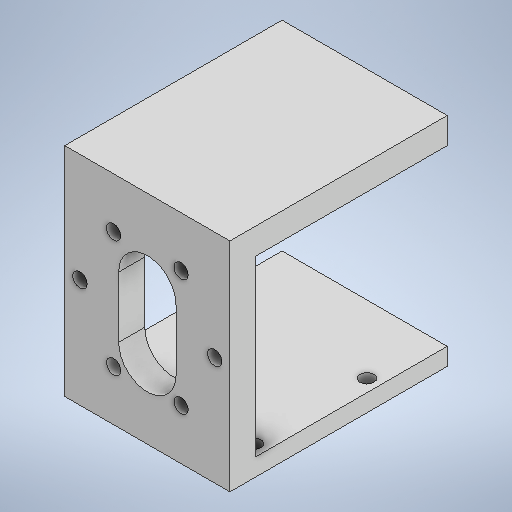
# Autodesk Inventor part: ギアボックス
Saved by Autodesk Inventor 2026.2 (Build 302298010, 298A)
## iProperties
Created: 2026-05-06
Part Number: ギアボックス
Material: 一般
Document SubType Name: Modeling
Designer: Yagis
Density: 1 g/cm^3
Appearance: 既定
Author: Yagis
Autodesk Inventor part; units mm, degrees
ref_plane "YZ Plane" through (0, 0, 0) normal (1, 0, 0) x (0, 1, 0)
ref_plane "XZ Plane" through (0, 0, 0) normal (0, 1, 0) x (-1, 0, 0)
ref_plane "XY Plane" through (0, 0, 0) normal (0, 0, 1) x (1, 0, 0)
sketch "スケッチ1" plane through (0, 0, 0) normal (0, 0, 1) x (1, 0, 0)
  line L0 (0, 0) -> (38, 0)
  line L1 (38, 0) -> (38, 24)
  line L2 (38, 24) -> (0, 24)
  line L3 (0, 24) -> (0, 0)
  line L4 (0, 4) -> (38, 4)
  line L5 (12.4, 31) -> (25.6, 31)
  line L6 (25.6, 31) -> (25.6, 17)
  line L7 (25.6, 17) -> (12.4, 17)
  line L8 (12.4, 17) -> (12.4, 31)
  arc A0 (25.6, 31) -> (12.4, 31) centre (19, 31) ccw
  arc A1 (12.4, 17) -> (25.6, 17) centre (19, 17) ccw
  line L9 (0, 24) -> (38, 24)
  line L10 (38, 24) -> (38, 44)
  line L11 (38, 44) -> (0, 44)
  line L12 (0, 44) -> (0, 24)
  line L13 (0, 44) -> (38, 44)
  line L14 (38, 44) -> (38, 50)
  line L15 (38, 50) -> (0, 50)
  line L16 (0, 50) -> (0, 44)
  point P0 (19, 24)
  point P1 (19, 39.6)
  point P2 (25.6, 24)
  point P3 (12.4, 24)
  dimension "d0" = 38
  dimension "d1" = 24
  dimension "d2" = 4
  dimension "d3" = 15.6
  dimension "d4" = 13.2
  dimension "d5" = 14
  dimension "d6" = 7
  dimension "d7" = 19
  dimension "d49" = 6
  dimension "d50" = 38
  dimension "d51" = 20
  dimension "d52" = 38
  constraints: 34 end point, 8 parallel, 5 perpendicular, 4 horizontal, 4 point on circle, 4 tangent, 2 centre point, 2 midpoint, 2 point on line
  measures "d0" distance of L0.start L0.end
  measures "d1" distance of L2.end L0.start
  measures "d2" distance between parallel lines of L0 L4
  measures "d3" distance of point (19, 24) point (19, 39.6)
  measures "d4" distance between parallel lines of L8 L6
  measures "d5" distance between parallel lines of L7 L5
  measures "d6" distance between parallel lines of L2 L7
  measures "d7" distance from line of L1 point (19, 17)
  measures "d49" distance between parallel lines of L13 L15
  measures "d50" distance between parallel lines of L12 L10
  measures "d51" distance between parallel lines of L11 L2
  measures "d52" distance between parallel lines of L16 L14
extrude "押し出し1" add sketch "スケッチ1" against normal blind 6 contours L3 L4 L1 L0 | L3 L2 L8 A1 L6 L1 L4 | L12 L11 L10 L2 L6 A0 L8 | L16 L15 L14 L11
extrude "押し出し2" add sketch "スケッチ1" against normal blind 50 contours L3 L4 L1 L0 | L16 L15 L14 L11
sketch "スケッチ2" plane through (0, 0, 0) normal (0, 0, 1) x (1, 0, 0)
  line L0 (0, 50) -> (0, 0) projected
  line L1 (38, 50) -> (0, 50) projected
  point P0 (3.5, 25)
  point P1 (19, 25)
  point P2 (11.25, 11.5766)
  point P3 (26.75, 11.5766)
  point P4 (34.5, 25)
  point P5 (26.75, 38.4234)
  point P6 (11.25, 38.4234)
  point P7 (0, 25)
  point P8 (19, 43.6)
  point P9 (0, 25)
  point P10 (19, 50)
  dimension "d16" = 360
  dimension "d18" = 15.5
  constraints: 3 horizontal alignment, 2 midpoint, 2 vertical alignment, 7 other
  measures "d18" distance of point (3.5, 25) point (19, 25)
hole "穴1" at (3.5, 25, 0) at (19, 25, 0) at (11.25, 11.5766, 0) at (26.75, 11.5766, 0) at (34.5, 25, 0) at (26.75, 38.4234, 0) at (11.25, 38.4234, 0) direction (0, 0, -1) diameter 3.3 depth 8.1 tip angle 118
sketch "スケッチ4" plane through (0, 4, -6) normal (0, 1, 0) x (1, 0, 0)
  point P0 (0, -6)
  point P1 (3.1531, 2.3812)
  point P2 (35.1531, 2.3812)
  point P3 (35.1531, 28.3812)
  point P4 (3.1531, 28.3812)
  dimension "d47" = 32
  dimension "d48" = 26
  constraints: 2 horizontal alignment, 2 vertical alignment
  measures "d47" distance of point (35.153, 2.381) point (3.153, 2.381)
  measures "d48" distance of point (35.153, 28.381) point (35.153, 2.381)
hole "穴3" at (3.1531, 4, -8.3812) at (35.1531, 4, -8.3812) at (35.1531, 4, -34.3812) at (3.1531, 4, -34.3812) direction (0, -1, 0) diameter 3.2 depth 8.1 tip angle 118
equation "\"d7\" = 0.5 * d0"
equation "\"d51\" = d1 - d2"
